Autodesk Inventor part; units mm, degrees
(part 4 of 4)
sketch "Двотавр 16" plane through (0, 0, 0) normal (0, 0, 1) x (1, 0, 0)
  arc A0 (264.3183, 276.423) -> (256.8007, 284.866) centre (255.8183, 276.423) ccw
  arc A1 (276.8359, 284.866) -> (269.3183, 276.423) centre (277.8183, 276.423) ccw
  arc A2 (256.8007, 143.1381) -> (264.3183, 151.5811) centre (255.8183, 151.5811) ccw
  arc A3 (269.3183, 151.5811) -> (276.8359, 143.1381) centre (277.8183, 151.5811) ccw
  line L0 (226.3183, 134.002) -> (307.3183, 134.002)
  line L1 (269.3183, 151.5811) -> (269.3183, 276.423)
  line L2 (307.3183, 294.002) -> (226.3183, 294.002)
  line L3 (264.3183, 276.423) -> (264.3183, 151.5811)
  line L4 (276.8359, 284.866) -> (304.4882, 288.0835)
  arc A4 (304.4882, 288.0835) -> (307.3183, 291.262) centre (304.1183, 291.262) ccw
  line L5 (307.3183, 291.262) -> (307.3183, 294.002)
  line L6 (256.8007, 284.866) -> (229.1485, 288.0835)
  arc A5 (226.3183, 291.262) -> (229.1485, 288.0835) centre (229.5183, 291.262) ccw
  line L7 (226.3183, 291.262) -> (226.3183, 294.002)
  line L8 (256.8007, 143.1381) -> (229.1485, 139.9206)
  arc A6 (229.1485, 139.9206) -> (226.3183, 136.742) centre (229.5183, 136.742) ccw
  line L9 (226.3183, 136.742) -> (226.3183, 134.002)
  line L10 (307.3183, 134.002) -> (307.3183, 136.742)
  arc A7 (307.3183, 136.742) -> (304.4882, 139.9206) centre (304.1183, 136.742) ccw
  line L11 (304.4882, 139.9206) -> (276.8359, 143.1381)
  point P0 (262.5027, 203.4372)
  point P1 (266.8183, 294.002)
  point P2 (266.8183, 134.002)
  point P3 (288.3183, 141.802)
  dimension "d1065" = 160
  dimension "d1066" = 81
  dimension "d1067" = 5
  dimension "d1068" = 8.5
  dimension "d1069" = 3.2
  dimension "d1070" = 2.74
  dimension "d1071" = 19
  dimension "d1072" = 7.8
  measures "d1065" distance between parallel lines of L0 L2
  measures "d1066" distance of L0.start L0.end
  measures "d1067" distance between parallel lines of L3 L1
  measures "d1068" radius of A3
  measures "d1069" radius of A7
  measures "d1070" distance of L0.end L10.end
  measures "d1071" horizontal distance of L0.end point (288.318, 141.802)
  measures "d1072" distance from line of L0 point (288.318, 141.802)
sketch "Двотавр 18" plane through (0, 0, 0) normal (0, 0, 1) x (1, 0, 0)
  arc A0 (264.4171, 285.6439) -> (256.3127, 294.5993) centre (255.4171, 285.6439) ccw
  arc A1 (277.6216, 294.5993) -> (269.5171, 285.6439) centre (278.5171, 285.6439) ccw
  arc A2 (256.3127, 133.4234) -> (264.4171, 142.3788) centre (255.4171, 142.3788) ccw
  arc A3 (269.5171, 142.3788) -> (277.6216, 133.4234) centre (278.5171, 142.3788) ccw
  line L0 (221.9671, 124.0114) -> (311.9671, 124.0114)
  line L1 (269.5171, 142.3788) -> (269.5171, 285.6439)
  line L2 (311.9671, 304.0114) -> (221.9671, 304.0114)
  line L3 (264.4171, 285.6439) -> (264.4171, 142.3788)
  line L4 (277.6216, 294.5993) -> (308.8154, 297.7187)
  arc A4 (308.8154, 297.7187) -> (311.9671, 301.2014) centre (308.4671, 301.2014) ccw
  line L5 (311.9671, 301.2014) -> (311.9671, 304.0114)
  line L6 (256.3127, 294.5993) -> (225.1189, 297.7187)
  arc A5 (221.9671, 301.2014) -> (225.1189, 297.7187) centre (225.4671, 301.2014) ccw
  line L7 (221.9671, 301.2014) -> (221.9671, 304.0114)
  line L8 (256.3127, 133.4234) -> (225.1189, 130.304)
  arc A6 (225.1189, 130.304) -> (221.9671, 126.8214) centre (225.4671, 126.8214) ccw
  line L9 (221.9671, 126.8214) -> (221.9671, 124.0114)
  line L10 (311.9671, 124.0114) -> (311.9671, 126.8214)
  arc A7 (311.9671, 126.8214) -> (308.8154, 130.304) centre (308.4671, 126.8214) ccw
  line L11 (308.8154, 130.304) -> (277.6216, 133.4234)
  point P0 (262.5027, 203.4372)
  point P1 (266.9671, 304.0114)
  point P2 (266.9671, 124.0114)
  point P3 (290.7421, 132.1114)
  dimension "d1073" = 180
  dimension "d1074" = 90
  dimension "d1075" = 5.1
  dimension "d1076" = 9
  dimension "d1077" = 3.5
  dimension "d1078" = 2.81
  dimension "d1079" = 21.225
  dimension "d1080" = 8.1
  measures "d1073" distance between parallel lines of L0 L2
  measures "d1074" distance of L0.start L0.end
  measures "d1075" distance between parallel lines of L3 L1
  measures "d1076" radius of A3
  measures "d1077" radius of A7
  measures "d1078" distance of L0.end L10.end
  measures "d1079" horizontal distance of L0.end point (290.742, 132.111)
  measures "d1080" distance from line of L0 point (290.742, 132.111)
sketch "Двотавр 18а" plane through (0, 0, 0) normal (0, 0, 1) x (1, 0, 0)
  arc A0 (317.1236, 126.8284) -> (313.9635, 130.3118) centre (313.6236, 126.8284) ccw
  line L0 (313.9635, 130.3118) -> (277.7996, 133.8404)
  arc A1 (269.6736, 142.7979) -> (277.7996, 133.8404) centre (278.6736, 142.7979) ccw
  arc A2 (256.4476, 133.8404) -> (264.5736, 142.7979) centre (255.5736, 142.7979) ccw
  line L1 (217.1236, 124.0184) -> (317.1236, 124.0184)
  line L2 (256.4476, 133.8404) -> (220.2837, 130.3118)
  line L3 (217.1236, 126.8284) -> (217.1236, 124.0184)
  arc A3 (220.2837, 130.3118) -> (217.1236, 126.8284) centre (220.6236, 126.8284) ccw
  line L4 (269.6736, 142.7979) -> (269.6736, 285.2389)
  line L5 (264.5736, 285.2389) -> (264.5736, 142.7979)
  arc A4 (264.5736, 285.2389) -> (256.4476, 294.1964) centre (255.5736, 285.2389) ccw
  arc A5 (277.7996, 294.1964) -> (269.6736, 285.2389) centre (278.6736, 285.2389) ccw
  line L6 (256.4476, 294.1964) -> (220.2837, 297.7249)
  arc A6 (217.1236, 301.2084) -> (220.2837, 297.7249) centre (220.6236, 301.2084) ccw
  line L7 (317.1236, 304.0184) -> (217.1236, 304.0184)
  line L8 (217.1236, 301.2084) -> (217.1236, 304.0184)
  line L9 (277.7996, 294.1964) -> (313.9635, 297.7249)
  arc A7 (313.9635, 297.7249) -> (317.1236, 301.2084) centre (313.6236, 301.2084) ccw
  line L10 (317.1236, 301.2084) -> (317.1236, 304.0184)
  line L11 (317.1236, 124.0184) -> (317.1236, 126.8284)
  point P0 (262.5027, 203.4372)
  point P1 (293.3986, 132.3184)
  point P2 (267.1236, 124.0184)
  point P3 (267.1236, 304.0184)
  dimension "d1081" = 180
  dimension "d1082" = 100
  dimension "d1083" = 5.1
  dimension "d1084" = 9
  dimension "d1085" = 3.5
  dimension "d1086" = 2.81
  dimension "d1087" = 23.725
  dimension "d1088" = 8.3
  measures "d1081" distance between parallel lines of L1 L7
  measures "d1082" distance of L1.start L11.start
  measures "d1083" distance between parallel lines of L5 L4
  measures "d1084" radius of A1
  measures "d1085" radius of A0
  measures "d1086" distance of L11.start L11.end
  measures "d1087" horizontal distance of L11.start point (293.399, 132.318)
  measures "d1088" distance from line of L1 point (293.399, 132.318)
sketch "Двотавр 20" plane through (0, 0, 0) normal (0, 0, 1) x (1, 0, 0)
  arc A0 (317.1239, 116.4425) -> (313.522, 120.4227) centre (313.1239, 116.4425) ccw
  line L0 (313.522, 120.4227) -> (278.2786, 123.9471)
  arc A1 (269.7239, 133.4) -> (278.2786, 123.9471) centre (279.2239, 133.4) ccw
  arc A2 (255.9692, 123.9471) -> (264.5239, 133.4) centre (255.0239, 133.4) ccw
  line L1 (217.1239, 114.0325) -> (317.1239, 114.0325)
  line L2 (255.9692, 123.9471) -> (220.7259, 120.4227)
  line L3 (217.1239, 116.4425) -> (217.1239, 114.0325)
  arc A3 (220.7259, 120.4227) -> (217.1239, 116.4425) centre (221.1239, 116.4425) ccw
  line L4 (269.7239, 133.4) -> (269.7239, 294.6651)
  line L5 (264.5239, 294.6651) -> (264.5239, 133.4)
  arc A4 (264.5239, 294.6651) -> (255.9692, 304.118) centre (255.0239, 294.6651) ccw
  arc A5 (278.2786, 304.118) -> (269.7239, 294.6651) centre (279.2239, 294.6651) ccw
  line L6 (255.9692, 304.118) -> (220.7259, 307.6424)
  arc A6 (217.1239, 311.6225) -> (220.7259, 307.6424) centre (221.1239, 311.6225) ccw
  line L7 (317.1239, 314.0325) -> (217.1239, 314.0325)
  line L8 (217.1239, 311.6225) -> (217.1239, 314.0325)
  line L9 (278.2786, 304.118) -> (313.522, 307.6424)
  arc A7 (313.522, 307.6424) -> (317.1239, 311.6225) centre (313.1239, 311.6225) ccw
  line L10 (317.1239, 311.6225) -> (317.1239, 314.0325)
  line L11 (317.1239, 114.0325) -> (317.1239, 116.4425)
  point P0 (262.5027, 203.4372)
  point P1 (293.4239, 122.4325)
  point P2 (267.1239, 114.0325)
  point P3 (267.1239, 314.0325)
  dimension "d1089" = 200
  dimension "d1090" = 100
  dimension "d1091" = 5.2
  dimension "d1092" = 9.5
  dimension "d1093" = 4
  dimension "d1094" = 2.41
  dimension "d1095" = 23.7
  dimension "d1096" = 8.4
  measures "d1089" distance between parallel lines of L1 L7
  measures "d1090" distance of L1.start L11.start
  measures "d1091" distance between parallel lines of L5 L4
  measures "d1092" radius of A1
  measures "d1093" radius of A0
  measures "d1094" distance of L11.start L11.end
  measures "d1095" horizontal distance of L11.start point (293.424, 122.433)
  measures "d1096" distance from line of L1 point (293.424, 122.433)
sketch "Двотавр 20а" plane through (0, 0, 0) normal (0, 0, 1) x (1, 0, 0)
  line L0 (322.2804, 114.0395) -> (322.2804, 116.4495)
  arc A0 (322.2804, 116.4495) -> (318.6697, 120.4306) centre (318.2804, 116.4495) ccw
  line L1 (318.6697, 120.4306) -> (278.4558, 124.363)
  arc A1 (269.8804, 133.8179) -> (278.4558, 124.363) centre (279.3804, 133.8179) ccw
  arc A2 (256.1049, 124.363) -> (264.6804, 133.8179) centre (255.1804, 133.8179) ccw
  line L2 (212.2804, 114.0395) -> (322.2804, 114.0395)
  line L3 (256.1049, 124.363) -> (215.8911, 120.4306)
  line L4 (212.2804, 116.4495) -> (212.2804, 114.0395)
  arc A3 (215.8911, 120.4306) -> (212.2804, 116.4495) centre (216.2804, 116.4495) ccw
  line L5 (269.8804, 133.8179) -> (269.8804, 294.2612)
  line L6 (264.6804, 294.2612) -> (264.6804, 133.8179)
  line L7 (256.1049, 303.7161) -> (215.8911, 307.6485)
  arc A4 (212.2804, 311.6295) -> (215.8911, 307.6485) centre (216.2804, 311.6295) ccw
  line L8 (212.2804, 311.6295) -> (212.2804, 314.0395)
  line L9 (322.2804, 314.0395) -> (212.2804, 314.0395)
  arc A5 (264.6804, 294.2612) -> (256.1049, 303.7161) centre (255.1804, 294.2612) ccw
  arc A6 (278.4558, 303.7161) -> (269.8804, 294.2612) centre (279.3804, 294.2612) ccw
  line L10 (278.4558, 303.7161) -> (318.6697, 307.6485)
  line L11 (322.2804, 311.6295) -> (322.2804, 314.0395)
  arc A7 (318.6697, 307.6485) -> (322.2804, 311.6295) centre (318.2804, 311.6295) ccw
  point P0 (262.5027, 203.4372)
  point P1 (296.0804, 122.6395)
  point P2 (267.2804, 114.0395)
  point P3 (267.2804, 314.0395)
  dimension "d1097" = 200
  dimension "d1098" = 110
  dimension "d1099" = 5.2
  dimension "d1100" = 9.5
  dimension "d1101" = 4
  dimension "d1102" = 2.41
  dimension "d1103" = 26.2
  dimension "d1104" = 8.6
  measures "d1097" distance between parallel lines of L2 L9
  measures "d1098" distance of L2.start L0.start
  measures "d1099" distance between parallel lines of L6 L5
  measures "d1100" radius of A1
  measures "d1101" radius of A0
  measures "d1102" distance of L0.start L0.end
  measures "d1103" horizontal distance of L0.start point (296.08, 122.64)
  measures "d1104" distance from line of L2 point (296.08, 122.64)
sketch "Двотавр 22" plane through (0, 0, 0) normal (0, 0, 1) x (1, 0, 0)
  line L0 (322.294, 104.0391) -> (322.294, 106.5091)
  arc A0 (322.294, 106.5091) -> (318.6912, 110.4893) centre (318.294, 106.5091) ccw
  line L1 (318.6912, 110.4893) -> (279.0012, 114.4496)
  arc A1 (269.994, 124.4002) -> (279.0012, 114.4496) centre (279.994, 124.4002) ccw
  arc A2 (255.5869, 114.4496) -> (264.594, 124.4002) centre (254.594, 124.4002) ccw
  line L2 (212.294, 104.0391) -> (322.294, 104.0391)
  line L3 (255.5869, 114.4496) -> (215.8969, 110.4893)
  line L4 (212.294, 106.5091) -> (212.294, 104.0391)
  arc A3 (215.8969, 110.4893) -> (212.294, 106.5091) centre (216.294, 106.5091) ccw
  line L5 (269.994, 124.4002) -> (269.994, 303.678)
  line L6 (264.594, 303.678) -> (264.594, 124.4002)
  line L7 (255.5869, 313.6286) -> (215.8969, 317.5889)
  arc A4 (212.294, 321.5691) -> (215.8969, 317.5889) centre (216.294, 321.5691) ccw
  line L8 (212.294, 321.5691) -> (212.294, 324.0391)
  line L9 (322.294, 324.0391) -> (212.294, 324.0391)
  arc A5 (264.594, 303.678) -> (255.5869, 313.6286) centre (254.594, 303.678) ccw
  arc A6 (279.0012, 313.6286) -> (269.994, 303.678) centre (279.994, 303.678) ccw
  line L10 (279.0012, 313.6286) -> (318.6912, 317.5889)
  line L11 (322.294, 321.5691) -> (322.294, 324.0391)
  arc A7 (318.6912, 317.5889) -> (322.294, 321.5691) centre (318.294, 321.5691) ccw
  point P0 (262.5027, 203.4372)
  point P1 (296.144, 112.7391)
  point P2 (267.294, 104.0391)
  point P3 (267.294, 324.0391)
  dimension "d1105" = 220
  dimension "d1106" = 110
  dimension "d1107" = 5.4
  dimension "d1108" = 10
  dimension "d1109" = 4
  dimension "d1110" = 2.47
  dimension "d1111" = 26.15
  dimension "d1112" = 8.7
  measures "d1105" distance between parallel lines of L2 L9
  measures "d1106" distance of L2.start L0.start
  measures "d1107" distance between parallel lines of L6 L5
  measures "d1108" radius of A1
  measures "d1109" radius of A0
  measures "d1110" distance of L0.start L0.end
  measures "d1111" horizontal distance of L0.start point (296.144, 112.739)
  measures "d1112" distance from line of L2 point (296.144, 112.739)
sketch "Двотавр 22а" plane through (0, 0, 0) normal (0, 0, 1) x (1, 0, 0)
  line L0 (327.4505, 104.0461) -> (327.4505, 106.5161)
  arc A0 (327.4505, 106.5161) -> (323.8398, 110.4971) centre (323.4505, 106.5161) ccw
  line L1 (323.8398, 110.4971) -> (279.1771, 114.8654)
  arc A1 (270.1505, 124.8179) -> (279.1771, 114.8654) centre (280.1505, 124.8179) ccw
  arc A2 (255.7239, 114.8654) -> (264.7505, 124.8179) centre (254.7505, 124.8179) ccw
  line L2 (207.4505, 104.0461) -> (327.4505, 104.0461)
  line L3 (255.7239, 114.8654) -> (211.0611, 110.4971)
  line L4 (207.4505, 106.5161) -> (207.4505, 104.0461)
  arc A3 (211.0611, 110.4971) -> (207.4505, 106.5161) centre (211.4505, 106.5161) ccw
  line L5 (264.7505, 303.2743) -> (264.7505, 124.8179)
  line L6 (270.1505, 124.8179) -> (270.1505, 303.2743)
  line L7 (279.1771, 313.2268) -> (323.8398, 317.5951)
  arc A4 (323.8398, 317.5951) -> (327.4505, 321.5761) centre (323.4505, 321.5761) ccw
  line L8 (327.4505, 321.5761) -> (327.4505, 324.0461)
  line L9 (327.4505, 324.0461) -> (207.4505, 324.0461)
  arc A5 (279.1771, 313.2268) -> (270.1505, 303.2743) centre (280.1505, 303.2743) ccw
  arc A6 (264.7505, 303.2743) -> (255.7239, 313.2268) centre (254.7505, 303.2743) ccw
  line L10 (255.7239, 313.2268) -> (211.0611, 317.5951)
  arc A7 (207.4505, 321.5761) -> (211.0611, 317.5951) centre (211.4505, 321.5761) ccw
  line L11 (207.4505, 321.5761) -> (207.4505, 324.0461)
  point P0 (262.5027, 203.4372)
  point P1 (298.8005, 112.9461)
  point P2 (267.4505, 104.0461)
  point P3 (267.4505, 324.0461)
  dimension "d1113" = 220
  dimension "d1114" = 120
  dimension "d1115" = 5.4
  dimension "d1116" = 10
  dimension "d1117" = 4
  dimension "d1118" = 2.47
  dimension "d1119" = 28.65
  dimension "d1120" = 8.9
  measures "d1113" distance between parallel lines of L2 L9
  measures "d1114" distance of L2.start L0.start
  measures "d1115" distance between parallel lines of L5 L6
  measures "d1116" radius of A1
  measures "d1117" radius of A0
  measures "d1118" distance of L0.start L0.end
  measures "d1119" horizontal distance of L0.start point (298.8, 112.946)
  measures "d1120" distance from line of L2 point (298.8, 112.946)
sketch "Двотавр 24" plane through (0, 0, 0) normal (0, 0, 1) x (1, 0, 0)
  line L0 (264.5861, 312.3079) -> (264.5861, 115.7752)
  line L1 (270.1861, 115.7752) -> (270.1861, 312.3079)
  line L2 (279.6435, 322.7561) -> (321.2833, 326.9114)
  arc A0 (321.2833, 326.9114) -> (324.8861, 330.8916) centre (320.8861, 330.8916) ccw
  line L3 (324.8861, 330.8916) -> (324.8861, 334.0416)
  line L4 (324.8861, 334.0416) -> (209.8861, 334.0416)
  arc A1 (279.6435, 322.7561) -> (270.1861, 312.3079) centre (280.6861, 312.3079) ccw
  arc A2 (264.5861, 312.3079) -> (255.1288, 322.7561) centre (254.0861, 312.3079) ccw
  line L5 (255.1288, 322.7561) -> (213.4889, 326.9114)
  arc A3 (209.8861, 330.8916) -> (213.4889, 326.9114) centre (213.8861, 330.8916) ccw
  line L6 (209.8861, 330.8916) -> (209.8861, 334.0416)
  line L7 (324.8861, 94.0416) -> (324.8861, 97.1916)
  arc A4 (324.8861, 97.1916) -> (321.2833, 101.1718) centre (320.8861, 97.1916) ccw
  line L8 (321.2833, 101.1718) -> (279.6435, 105.3271)
  arc A5 (255.1288, 105.3271) -> (264.5861, 115.7752) centre (254.0861, 115.7752) ccw
  line L9 (209.8861, 94.0416) -> (324.8861, 94.0416)
  arc A6 (270.1861, 115.7752) -> (279.6435, 105.3271) centre (280.6861, 115.7752) ccw
  line L10 (255.1288, 105.3271) -> (213.4889, 101.1718)
  arc A7 (213.4889, 101.1718) -> (209.8861, 97.1916) centre (213.8861, 97.1916) ccw
  line L11 (209.8861, 97.1916) -> (209.8861, 94.0416)
  point P0 (262.5027, 203.4372)
  point P1 (267.3861, 334.0416)
  point P2 (297.5361, 103.5416)
  point P3 (267.3861, 94.0416)
  dimension "d1121" = 240
  dimension "d1122" = 115
  dimension "d1123" = 5.6
  dimension "d1124" = 10.5
  dimension "d1125" = 4
  dimension "d1126" = 3.15
  dimension "d1127" = 27.35
  dimension "d1128" = 9.5
  measures "d1121" distance between parallel lines of L9 L4
  measures "d1122" distance of L9.start L9.end
  measures "d1123" distance between parallel lines of L0 L1
  measures "d1124" radius of A6
  measures "d1125" radius of A4
  measures "d1126" distance of L9.end L7.end
  measures "d1127" horizontal distance of L9.end point (297.536, 103.542)
  measures "d1128" distance from line of L9 point (297.536, 103.542)
sketch "Двотавр 24а" plane through (0, 0, 0) normal (0, 0, 1) x (1, 0, 0)
  line L0 (255.3043, 105.9275) -> (208.637, 101.1807)
  arc A0 (208.637, 101.1807) -> (205.0418, 97.2013) centre (209.0418, 97.2013) ccw
  line L1 (205.0418, 94.0513) -> (330.0418, 94.0513)
  line L2 (205.0418, 97.2013) -> (205.0418, 94.0513)
  arc A1 (255.3043, 105.9275) -> (264.7418, 116.3736) centre (254.2418, 116.3736) ccw
  arc A2 (270.3418, 116.3736) -> (279.7793, 105.9275) centre (280.8418, 116.3736) ccw
  line L3 (326.4466, 101.1807) -> (279.7793, 105.9275)
  line L4 (330.0418, 94.0513) -> (330.0418, 97.2013)
  arc A3 (330.0418, 97.2013) -> (326.4466, 101.1807) centre (326.0418, 97.2013) ccw
  line L5 (264.7418, 311.7289) -> (264.7418, 116.3736)
  line L6 (270.3418, 116.3736) -> (270.3418, 311.7289)
  line L7 (279.7793, 322.175) -> (326.4466, 326.9218)
  arc A4 (326.4466, 326.9218) -> (330.0418, 330.9013) centre (326.0418, 330.9013) ccw
  line L8 (330.0418, 330.9013) -> (330.0418, 334.0513)
  arc A5 (279.7793, 322.175) -> (270.3418, 311.7289) centre (280.8418, 311.7289) ccw
  arc A6 (264.7418, 311.7289) -> (255.3043, 322.175) centre (254.2418, 311.7289) ccw
  line L9 (330.0418, 334.0513) -> (205.0418, 334.0513)
  line L10 (255.3043, 322.175) -> (208.637, 326.9218)
  arc A7 (205.0418, 330.9013) -> (208.637, 326.9218) centre (209.0418, 330.9013) ccw
  line L11 (205.0418, 330.9013) -> (205.0418, 334.0513)
  point P0 (262.5027, 203.4372)
  point P1 (267.5418, 94.0513)
  point P2 (300.1918, 103.8513)
  point P3 (267.5418, 334.0513)
  dimension "d1129" = 240
  dimension "d1130" = 125
  dimension "d1131" = 5.6
  dimension "d1132" = 10.5
  dimension "d1133" = 4
  dimension "d1134" = 3.15
  dimension "d1135" = 29.85
  dimension "d1136" = 9.8
  measures "d1129" distance between parallel lines of L1 L9
  measures "d1130" distance of L1.start L1.end
  measures "d1131" distance between parallel lines of L5 L6
  measures "d1132" radius of A2
  measures "d1133" radius of A3
  measures "d1134" distance of L1.end L4.end
  measures "d1135" horizontal distance of L1.end point (300.192, 103.851)
  measures "d1136" distance from line of L1 point (300.192, 103.851)
sketch "Двотавр 27" plane through (0, 0, 0) normal (0, 0, 1) x (1, 0, 0)
  line L0 (254.6336, 90.843) -> (209.0957, 86.3024)
  arc A0 (209.0957, 86.3024) -> (205.0422, 81.8246) centre (209.5422, 81.8246) ccw
  line L1 (205.0422, 79.0646) -> (330.0422, 79.0646)
  line L2 (205.0422, 81.8246) -> (205.0422, 79.0646)
  arc A1 (254.6336, 90.843) -> (264.5422, 101.7887) centre (253.5422, 101.7887) ccw
  arc A2 (270.5422, 101.7887) -> (280.4508, 90.843) centre (281.5422, 101.7887) ccw
  line L3 (325.9887, 86.3024) -> (280.4508, 90.843)
  line L4 (330.0422, 79.0646) -> (330.0422, 81.8246)
  arc A3 (330.0422, 81.8246) -> (325.9887, 86.3024) centre (325.5422, 81.8246) ccw
  line L5 (264.5422, 326.3405) -> (264.5422, 101.7887)
  line L6 (270.5422, 101.7887) -> (270.5422, 326.3405)
  line L7 (280.4508, 337.2862) -> (325.9887, 341.8268)
  arc A4 (325.9887, 341.8268) -> (330.0422, 346.3046) centre (325.5422, 346.3046) ccw
  line L8 (330.0422, 346.3046) -> (330.0422, 349.0646)
  arc A5 (280.4508, 337.2862) -> (270.5422, 326.3405) centre (281.5422, 326.3405) ccw
  arc A6 (264.5422, 326.3405) -> (254.6336, 337.2862) centre (253.5422, 326.3405) ccw
  line L9 (330.0422, 349.0646) -> (205.0422, 349.0646)
  line L10 (254.6336, 337.2862) -> (209.0957, 341.8268)
  arc A7 (205.0422, 346.3046) -> (209.0957, 341.8268) centre (209.5422, 346.3046) ccw
  line L11 (205.0422, 346.3046) -> (205.0422, 349.0646)
  point P0 (262.5027, 203.4372)
  point P1 (267.5422, 79.0646)
  point P2 (300.2922, 88.8646)
  point P3 (267.5422, 349.0646)
  dimension "d1137" = 270
  dimension "d1138" = 125
  dimension "d1139" = 6
  dimension "d1140" = 11
  dimension "d1141" = 4.5
  dimension "d1142" = 2.76
  dimension "d1143" = 29.75
  dimension "d1144" = 9.8
  measures "d1137" distance between parallel lines of L1 L9
  measures "d1138" distance of L1.start L1.end
  measures "d1139" distance between parallel lines of L5 L6
  measures "d1140" radius of A2
  measures "d1141" radius of A3
  measures "d1142" distance of L1.end L4.end
  measures "d1143" horizontal distance of L1.end point (300.292, 88.865)
  measures "d1144" distance from line of L1 point (300.292, 88.865)
sketch "Двотавр 27а" plane through (0, 0, 0) normal (0, 0, 1) x (1, 0, 0)
  line L0 (254.8464, 91.6302) -> (204.227, 86.3124)
  arc A0 (204.227, 86.3124) -> (200.1971, 81.8371) centre (204.6971, 81.8371) ccw
  line L1 (200.1971, 79.0771) -> (335.1971, 79.0771)
  line L2 (200.1971, 81.8371) -> (200.1971, 79.0771)
  arc A1 (254.8464, 91.6302) -> (264.6971, 102.57) centre (253.6971, 102.57) ccw
  arc A2 (270.6971, 102.57) -> (280.5479, 91.6302) centre (281.6971, 102.57) ccw
  line L3 (331.1673, 86.3124) -> (280.5479, 91.6302)
  arc A3 (335.1971, 81.8371) -> (331.1673, 86.3124) centre (330.6971, 81.8371) ccw
  line L4 (335.1971, 79.0771) -> (335.1971, 81.8371)
  line L5 (270.6971, 102.57) -> (270.6971, 325.5841)
  line L6 (264.6971, 325.5841) -> (264.6971, 102.57)
  arc A4 (280.5479, 336.5239) -> (270.6971, 325.5841) centre (281.6971, 325.5841) ccw
  line L7 (280.5479, 336.5239) -> (331.1673, 341.8417)
  arc A5 (331.1673, 341.8417) -> (335.1971, 346.3171) centre (330.6971, 346.3171) ccw
  line L8 (335.1971, 346.3171) -> (335.1971, 349.0771)
  line L9 (335.1971, 349.0771) -> (200.1971, 349.0771)
  line L10 (254.8464, 336.5239) -> (204.227, 341.8417)
  arc A6 (200.1971, 346.3171) -> (204.227, 341.8417) centre (204.6971, 346.3171) ccw
  line L11 (200.1971, 346.3171) -> (200.1971, 349.0771)
  arc A7 (264.6971, 325.5841) -> (254.8464, 336.5239) centre (253.6971, 325.5841) ccw
  point P0 (262.5027, 203.4372)
  point P1 (267.6971, 79.0771)
  point P2 (302.9471, 89.2771)
  point P3 (267.6971, 349.0771)
  dimension "d1153" = 270
  dimension "d1154" = 135
  dimension "d1155" = 6
  dimension "d1156" = 11
  dimension "d1157" = 4.5
  dimension "d1158" = 2.76
  dimension "d1159" = 32.25
  dimension "d1160" = 10.2
  measures "d1153" distance between parallel lines of L1 L9
  measures "d1154" distance of L1.start L4.start
  measures "d1155" distance between parallel lines of L6 L5
  measures "d1156" radius of A2
  measures "d1157" radius of A3
  measures "d1158" distance of L4.start L4.end
  measures "d1159" horizontal distance of L4.start point (302.947, 89.277)
  measures "d1160" distance from line of L1 point (302.947, 89.277)
sketch "Двотавр 30" plane through (0, 0, 0) normal (0, 0, 1) x (1, 0, 0)
  line L0 (253.6531, 76.412) -> (204.7161, 71.5315)
  arc A0 (204.7161, 71.5315) -> (200.2123, 66.5562) centre (205.2123, 66.5562) ccw
  line L1 (200.2123, 64.0862) -> (335.2123, 64.0862)
  line L2 (200.2123, 66.5562) -> (200.2123, 64.0862)
  arc A1 (253.6531, 76.412) -> (264.4623, 88.3528) centre (252.4623, 88.3528) ccw
  arc A2 (270.9623, 88.3528) -> (281.7714, 76.412) centre (282.9623, 88.3528) ccw
  line L3 (330.7085, 71.5315) -> (281.7714, 76.412)
  arc A3 (335.2123, 66.5562) -> (330.7085, 71.5315) centre (330.2123, 66.5562) ccw
  line L4 (335.2123, 64.0862) -> (335.2123, 66.5562)
  line L5 (270.9623, 88.3528) -> (270.9623, 339.8196)
  line L6 (264.4623, 339.8196) -> (264.4623, 88.3528)
  arc A4 (281.7714, 351.7603) -> (270.9623, 339.8196) centre (282.9623, 339.8196) ccw
  line L7 (281.7714, 351.7603) -> (330.7085, 356.6408)
  arc A5 (330.7085, 356.6408) -> (335.2123, 361.6162) centre (330.2123, 361.6162) ccw
  line L8 (335.2123, 361.6162) -> (335.2123, 364.0862)
  line L9 (335.2123, 364.0862) -> (200.2123, 364.0862)
  line L10 (253.6531, 351.7603) -> (204.7161, 356.6408)
  arc A6 (200.2123, 361.6162) -> (204.7161, 356.6408) centre (205.2123, 361.6162) ccw
  line L11 (200.2123, 361.6162) -> (200.2123, 364.0862)
  arc A7 (264.4623, 339.8196) -> (253.6531, 351.7603) centre (252.4623, 339.8196) ccw
  point P0 (262.5027, 203.4372)
  point P1 (267.7123, 64.0862)
  point P2 (303.0873, 74.2862)
  point P3 (267.7123, 364.0862)
  dimension "d1161" = 300
  dimension "d1162" = 135
  dimension "d1163" = 6.5
  dimension "d1164" = 12
  dimension "d1165" = 5
  dimension "d1166" = 2.47
  dimension "d1167" = 32.125
  dimension "d1168" = 10.2
  measures "d1161" distance between parallel lines of L1 L9
  measures "d1162" distance of L1.start L4.start
  measures "d1163" distance between parallel lines of L6 L5
  measures "d1164" radius of A2
  measures "d1165" radius of A3
  measures "d1166" distance of L4.start L4.end
  measures "d1167" horizontal distance of L4.start point (303.087, 74.286)
  measures "d1168" distance from line of L1 point (303.087, 74.286)
sketch "Двотавр 30а" plane through (0, 0, 0) normal (0, 0, 1) x (1, 0, 0)
  line L0 (340.3665, 64.1013) -> (340.3665, 66.5713)
  arc A0 (340.3665, 66.5713) -> (335.9036, 71.5424) centre (335.3665, 66.5713) ccw
  arc A1 (281.8275, 350.8175) -> (271.1165, 338.8869) centre (283.1165, 338.8869) ccw
  arc A2 (264.6165, 338.8869) -> (253.9056, 350.8175) centre (252.6165, 338.8869) ccw
  line L1 (281.8275, 350.8175) -> (335.9036, 356.6602)
  arc A3 (335.9036, 356.6602) -> (340.3665, 361.6313) centre (335.3665, 361.6313) ccw
  line L2 (340.3665, 361.6313) -> (340.3665, 364.1013)
  line L3 (340.3665, 364.1013) -> (195.3665, 364.1013)
  line L4 (253.9056, 350.8175) -> (199.8294, 356.6602)
  arc A4 (195.3665, 361.6313) -> (199.8294, 356.6602) centre (200.3665, 361.6313) ccw
  line L5 (195.3665, 361.6313) -> (195.3665, 364.1013)
  line L6 (335.9036, 71.5424) -> (281.8275, 77.3852)
  arc A5 (271.1165, 89.3157) -> (281.8275, 77.3852) centre (283.1165, 89.3157) ccw
  arc A6 (253.9056, 77.3852) -> (264.6165, 89.3157) centre (252.6165, 89.3157) ccw
  line L7 (195.3665, 64.1013) -> (340.3665, 64.1013)
  line L8 (253.9056, 77.3852) -> (199.8294, 71.5424)
  line L9 (195.3665, 66.5713) -> (195.3665, 64.1013)
  arc A7 (199.8294, 71.5424) -> (195.3665, 66.5713) centre (200.3665, 66.5713) ccw
  line L10 (271.1165, 89.3157) -> (271.1165, 338.8869)
  line L11 (264.6165, 338.8869) -> (264.6165, 89.3157)
  point P0 (262.5027, 203.4372)
  point P1 (267.8665, 364.1013)
  point P2 (305.7415, 74.8013)
  point P3 (267.8665, 64.1013)
  dimension "d1169" = 300
  dimension "d1170" = 145
  dimension "d1171" = 6.5
  dimension "d1172" = 12
  dimension "d1173" = 5
  dimension "d1174" = 2.47
  dimension "d1175" = 34.625
  dimension "d1176" = 10.7
  measures "d1169" distance between parallel lines of L7 L3
  measures "d1170" distance of L7.start L0.start
  measures "d1171" distance between parallel lines of L11 L10
  measures "d1172" radius of A5
  measures "d1173" radius of A0
  measures "d1174" distance of L0.start L0.end
  measures "d1175" horizontal distance of L0.start point (305.742, 74.801)
  measures "d1176" distance from line of L7 point (305.742, 74.801)
sketch "Двотавр 33" plane through (0, 0, 0) normal (0, 0, 1) x (1, 0, 0)
  line L0 (337.8184, 49.0868) -> (337.8184, 52.4468)
  arc A0 (337.8184, 52.4468) -> (333.3142, 57.4222) centre (332.8184, 52.4468) ccw
  arc A1 (283.0293, 365.7404) -> (271.3184, 352.8045) centre (284.3184, 352.8045) ccw
  arc A2 (264.3184, 352.8045) -> (252.6075, 365.7404) centre (251.3184, 352.8045) ccw
  line L1 (283.0293, 365.7404) -> (333.3142, 370.7515)
  arc A3 (333.3142, 370.7515) -> (337.8184, 375.7268) centre (332.8184, 375.7268) ccw
  line L2 (337.8184, 375.7268) -> (337.8184, 379.0868)
  line L3 (337.8184, 379.0868) -> (197.8184, 379.0868)
  line L4 (252.6075, 365.7404) -> (202.3226, 370.7515)
  arc A4 (197.8184, 375.7268) -> (202.3226, 370.7515) centre (202.8184, 375.7268) ccw
  line L5 (197.8184, 375.7268) -> (197.8184, 379.0868)
  line L6 (333.3142, 57.4222) -> (283.0293, 62.4333)
  arc A5 (271.3184, 75.3692) -> (283.0293, 62.4333) centre (284.3184, 75.3692) ccw
  arc A6 (252.6075, 62.4333) -> (264.3184, 75.3692) centre (251.3184, 75.3692) ccw
  line L7 (197.8184, 49.0868) -> (337.8184, 49.0868)
  line L8 (252.6075, 62.4333) -> (202.3226, 57.4222)
  line L9 (197.8184, 52.4468) -> (197.8184, 49.0868)
  arc A7 (202.3226, 57.4222) -> (197.8184, 52.4468) centre (202.8184, 52.4468) ccw
  line L10 (271.3184, 75.3692) -> (271.3184, 352.8045)
  line L11 (264.3184, 352.8045) -> (264.3184, 75.3692)
  point P0 (262.5027, 203.4372)
  point P1 (267.8184, 379.0868)
  point P2 (304.5684, 60.2868)
  point P3 (267.8184, 49.0868)
  dimension "d1177" = 330
  dimension "d1178" = 140
  dimension "d1179" = 7
  dimension "d1180" = 13
  dimension "d1181" = 5
  dimension "d1182" = 3.36
  dimension "d1183" = 33.25
  dimension "d1184" = 11.2
  measures "d1177" distance between parallel lines of L7 L3
  measures "d1178" distance of L7.start L0.start
  measures "d1179" distance between parallel lines of L11 L10
  measures "d1180" radius of A5
  measures "d1181" radius of A0
  measures "d1182" distance of L0.start L0.end
  measures "d1183" horizontal distance of L0.start point (304.568, 60.287)
  measures "d1184" distance from line of L7 point (304.568, 60.287)
sketch "Двотавр 36" plane through (0, 0, 0) normal (0, 0, 1) x (1, 0, 0)
  line L0 (340.3964, 34.1209) -> (340.3964, 37.5609)
  arc A0 (340.3964, 37.5609) -> (334.9919, 43.5312) centre (334.3964, 37.5609) ccw
  arc A1 (284.2568, 379.65) -> (271.6464, 365.7191) centre (285.6464, 365.7191) ccw
  arc A2 (264.1464, 365.7191) -> (251.5359, 379.65) centre (250.1464, 365.7191) ccw
  line L1 (284.2568, 379.65) -> (334.9919, 384.7105)
  arc A3 (334.9919, 384.7105) -> (340.3964, 390.6809) centre (334.3964, 390.6809) ccw
  line L2 (340.3964, 390.6809) -> (340.3964, 394.1209)
  line L3 (340.3964, 394.1209) -> (195.3964, 394.1209)
  line L4 (251.5359, 379.65) -> (200.8009, 384.7105)
  arc A4 (195.3964, 390.6809) -> (200.8009, 384.7105) centre (201.3964, 390.6809) ccw
  line L5 (195.3964, 390.6809) -> (195.3964, 394.1209)
  line L6 (334.9919, 43.5312) -> (284.2568, 48.5917)
  arc A5 (271.6464, 62.5226) -> (284.2568, 48.5917) centre (285.6464, 62.5226) ccw
  arc A6 (251.5359, 48.5917) -> (264.1464, 62.5226) centre (250.1464, 62.5226) ccw
  line L7 (195.3964, 34.1209) -> (340.3964, 34.1209)
  line L8 (251.5359, 48.5917) -> (200.8009, 43.5312)
  line L9 (195.3964, 37.5609) -> (195.3964, 34.1209)
  arc A7 (200.8009, 43.5312) -> (195.3964, 37.5609) centre (201.3964, 37.5609) ccw
  line L10 (271.6464, 62.5226) -> (271.6464, 365.7191)
  line L11 (264.1464, 365.7191) -> (264.1464, 62.5226)
  point P0 (262.5027, 203.4372)
  point P1 (267.8964, 394.1209)
  point P2 (306.0214, 46.4209)
  point P3 (267.8964, 34.1209)
  dimension "d1185" = 360
  dimension "d1186" = 145
  dimension "d1187" = 7.5
  dimension "d1188" = 14
  dimension "d1189" = 6
  dimension "d1190" = 3.44
  dimension "d1191" = 34.375
  dimension "d1192" = 12.3
  measures "d1185" distance between parallel lines of L7 L3
  measures "d1186" distance of L7.start L0.start
  measures "d1187" distance between parallel lines of L11 L10
  measures "d1188" radius of A5
  measures "d1189" radius of A0
  measures "d1190" distance of L0.start L0.end
  measures "d1191" horizontal distance of L0.start point (306.021, 46.421)
  measures "d1192" distance from line of L7 point (306.021, 46.421)
sketch "Двотавр 40" plane through (0, 0, 0) normal (0, 0, 1) x (1, 0, 0)
  line L0 (345.5809, 14.1255) -> (345.5809, 18.0355)
  arc A0 (345.5809, 18.0355) -> (340.1765, 24.0059) centre (339.5809, 18.0355) ccw
  arc A1 (285.7418, 398.8146) -> (272.2309, 383.8887) centre (287.2309, 383.8887) ccw
  arc A2 (263.9309, 383.8887) -> (250.4199, 398.8146) centre (248.9309, 383.8887) ccw
  line L1 (285.7418, 398.8146) -> (340.1765, 404.2451)
  arc A3 (340.1765, 404.2451) -> (345.5809, 410.2155) centre (339.5809, 410.2155) ccw
  line L2 (345.5809, 410.2155) -> (345.5809, 414.1255)
  line L3 (345.5809, 414.1255) -> (190.5809, 414.1255)
  line L4 (250.4199, 398.8146) -> (195.9852, 404.2451)
  arc A4 (190.5809, 410.2155) -> (195.9852, 404.2451) centre (196.5809, 410.2155) ccw
  line L5 (190.5809, 410.2155) -> (190.5809, 414.1255)
  line L6 (340.1765, 24.0059) -> (285.7418, 29.4364)
  arc A5 (272.2309, 44.3623) -> (285.7418, 29.4364) centre (287.2309, 44.3623) ccw
  arc A6 (250.4199, 29.4364) -> (263.9309, 44.3623) centre (248.9309, 44.3623) ccw
  line L7 (190.5809, 14.1255) -> (345.5809, 14.1255)
  line L8 (250.4199, 29.4364) -> (195.9852, 24.0059)
  line L9 (190.5809, 18.0355) -> (190.5809, 14.1255)
  arc A7 (195.9852, 24.0059) -> (190.5809, 18.0355) centre (196.5809, 18.0355) ccw
  line L10 (272.2309, 44.3623) -> (272.2309, 383.8887)
  line L11 (263.9309, 383.8887) -> (263.9309, 44.3623)
  point P0 (262.5027, 203.4372)
  point P1 (268.0809, 414.1255)
  point P2 (308.9059, 27.1255)
  point P3 (268.0809, 14.1255)
  dimension "d1193" = 400
  dimension "d1194" = 155
  dimension "d1195" = 8.3
  dimension "d1196" = 15
  dimension "d1197" = 6
  dimension "d1198" = 3.91
  dimension "d1199" = 36.675
  dimension "d1200" = 13
  measures "d1193" distance between parallel lines of L7 L3
  measures "d1194" distance of L7.start L0.start
  measures "d1195" distance between parallel lines of L11 L10
  measures "d1196" radius of A5
  measures "d1197" radius of A0
  measures "d1198" distance of L0.start L0.end
  measures "d1199" horizontal distance of L0.start point (308.906, 27.125)
  measures "d1200" distance from line of L7 point (308.906, 27.125)
sketch "Двотавр 45" plane through (0, 0, 0) normal (0, 0, 1) x (1, 0, 0)
  line L0 (348.1589, -10.8408) -> (348.1589, -6.7408)
  arc A0 (287.0718, 422.6329) -> (272.6589, 406.7118) centre (288.6589, 406.7118) ccw
  arc A1 (263.6589, 406.7118) -> (249.246, 422.6329) centre (247.6589, 406.7118) ccw
  line L1 (287.0718, 422.6329) -> (341.8533, 428.0937)
  arc A2 (341.8533, 428.0937) -> (348.1589, 435.0592) centre (341.1589, 435.0592) ccw
  line L2 (348.1589, 435.0592) -> (348.1589, 439.1592)
  line L3 (348.1589, 439.1592) -> (188.1589, 439.1592)
  line L4 (249.246, 422.6329) -> (194.4645, 428.0937)
  arc A3 (188.1589, 435.0592) -> (194.4645, 428.0937) centre (195.1589, 435.0592) ccw
  line L5 (188.1589, 435.0592) -> (188.1589, 439.1592)
  arc A4 (348.1589, -6.7408) -> (341.8533, 0.2247) centre (341.1589, -6.7408) ccw
  line L6 (341.8533, 0.2247) -> (287.0718, 5.6856)
  arc A5 (272.6589, 21.6067) -> (287.0718, 5.6856) centre (288.6589, 21.6067) ccw
  arc A6 (249.246, 5.6856) -> (263.6589, 21.6067) centre (247.6589, 21.6067) ccw
  line L7 (188.1589, -10.8408) -> (348.1589, -10.8408)
  line L8 (188.1589, -6.7408) -> (188.1589, -10.8408)
  arc A7 (194.4645, 0.2247) -> (188.1589, -6.7408) centre (195.1589, -6.7408) ccw
  line L9 (272.6589, 21.6067) -> (272.6589, 406.7118)
  line L10 (263.6589, 406.7118) -> (263.6589, 21.6067)
  line L11 (249.246, 5.6856) -> (194.4645, 0.2247)
  point P0 (262.5027, 203.4372)
  point P1 (268.1589, 439.1592)
  point P2 (310.4089, 3.3592)
  point P3 (268.1589, -10.8408)
  dimension "d1201" = 450
  dimension "d1202" = 160
  dimension "d1203" = 9
  dimension "d1204" = 16
  dimension "d1205" = 7
  dimension "d1206" = 4.1
  dimension "d1207" = 37.75
  dimension "d1208" = 14.2
  measures "d1201" distance between parallel lines of L7 L3
  measures "d1202" distance of L8.end L0.start
  measures "d1203" distance between parallel lines of L10 L9
  measures "d1204" radius of A5
  measures "d1205" radius of A4
  measures "d1206" distance of L0.start L0.end
  measures "d1207" horizontal distance of L0.start point (310.409, 3.359)
  measures "d1208" distance from line of L7 point (310.409, 3.359)
sketch "Двотавр 50" plane through (0, 0, 0) normal (0, 0, 1) x (1, 0, 0)
  line L0 (353.3429, -35.8362) -> (353.3429, -30.9662)
  arc A0 (288.6538, 446.4985) -> (273.3429, 429.5827) centre (290.3429, 429.5827) ccw
  arc A1 (263.3429, 429.5827) -> (248.032, 446.4985) centre (246.3429, 429.5827) ccw
  line L1 (288.6538, 446.4985) -> (347.0384, 452.3285)
  arc A2 (347.0384, 452.3285) -> (353.3429, 459.2938) centre (346.3429, 459.2938) ccw
  line L2 (353.3429, 459.2938) -> (353.3429, 464.1638)
  line L3 (353.3429, 464.1638) -> (183.3429, 464.1638)
  line L4 (248.032, 446.4985) -> (189.6474, 452.3285)
  arc A3 (183.3429, 459.2938) -> (189.6474, 452.3285) centre (190.3429, 459.2938) ccw
  line L5 (183.3429, 459.2938) -> (183.3429, 464.1638)
  arc A4 (353.3429, -30.9662) -> (347.0384, -24.0008) centre (346.3429, -30.9662) ccw
  line L6 (347.0384, -24.0008) -> (288.6538, -18.1708)
  arc A5 (273.3429, -1.255) -> (288.6538, -18.1708) centre (290.3429, -1.255) ccw
  arc A6 (248.032, -18.1708) -> (263.3429, -1.255) centre (246.3429, -1.255) ccw
  line L7 (183.3429, -35.8362) -> (353.3429, -35.8362)
  line L8 (183.3429, -30.9662) -> (183.3429, -35.8362)
  arc A7 (189.6474, -24.0008) -> (183.3429, -30.9662) centre (190.3429, -30.9662) ccw
  line L9 (273.3429, -1.255) -> (273.3429, 429.5827)
  line L10 (263.3429, 429.5827) -> (263.3429, -1.255)
  line L11 (248.032, -18.1708) -> (189.6474, -24.0008)
  point P0 (262.5027, 203.4372)
  point P1 (268.3429, 464.1638)
  point P2 (313.3429, -20.6362)
  point P3 (268.3429, -35.8362)
  dimension "d1209" = 500
  dimension "d1210" = 170
  dimension "d1211" = 10
  dimension "d1212" = 17
  dimension "d1213" = 7
  dimension "d1214" = 4.87
  dimension "d1215" = 40
  dimension "d1216" = 15.2
  measures "d1209" distance between parallel lines of L7 L3
  measures "d1210" distance of L8.end L0.start
  measures "d1211" distance between parallel lines of L10 L9
  measures "d1212" radius of A5
  measures "d1213" radius of A4
  measures "d1214" distance of L0.start L0.end
  measures "d1215" horizontal distance of L0.start point (313.343, -20.636)
  measures "d1216" distance from line of L7 point (313.343, -20.636)
sketch "Двотавр 55" plane through (0, 0, 0) normal (0, 0, 1) x (1, 0, 0)
  line L0 (358.5274, -60.8318) -> (358.5274, -54.8818)
  arc A0 (290.2413, 470.0717) -> (274.0274, 452.1606) centre (292.0274, 452.1606) ccw
  arc A1 (263.0274, 452.1606) -> (246.8136, 470.0717) centre (245.0274, 452.1606) ccw
  line L1 (290.2413, 470.0717) -> (352.2221, 476.2527)
  arc A2 (352.2221, 476.2527) -> (358.5274, 483.2182) centre (351.5274, 483.2182) ccw
  line L2 (358.5274, 483.2182) -> (358.5274, 489.1682)
  line L3 (358.5274, 489.1682) -> (178.5274, 489.1682)
  line L4 (246.8136, 470.0717) -> (184.8328, 476.2527)
  arc A3 (178.5274, 483.2182) -> (184.8328, 476.2527) centre (185.5274, 483.2182) ccw
  line L5 (178.5274, 483.2182) -> (178.5274, 489.1682)
  arc A4 (358.5274, -54.8818) -> (352.2221, -47.9164) centre (351.5274, -54.8818) ccw
  line L6 (352.2221, -47.9164) -> (290.2413, -41.7354)
  arc A5 (274.0274, -23.8242) -> (290.2413, -41.7354) centre (292.0274, -23.8242) ccw
  arc A6 (246.8136, -41.7354) -> (263.0274, -23.8242) centre (245.0274, -23.8242) ccw
  line L7 (178.5274, -60.8318) -> (358.5274, -60.8318)
  line L8 (178.5274, -54.8818) -> (178.5274, -60.8318)
  arc A7 (184.8328, -47.9164) -> (178.5274, -54.8818) centre (185.5274, -54.8818) ccw
  line L9 (274.0274, -23.8242) -> (274.0274, 452.1606)
  line L10 (263.0274, 452.1606) -> (263.0274, -23.8242)
  line L11 (246.8136, -41.7354) -> (184.8328, -47.9164)
  point P0 (262.5027, 203.4372)
  point P1 (268.5274, 489.1682)
  point P2 (316.2774, -44.3318)
  point P3 (268.5274, -60.8318)
  dimension "d1217" = 550
  dimension "d1218" = 180
  dimension "d1219" = 11
  dimension "d1220" = 18
  dimension "d1221" = 7
  dimension "d1222" = 5.95
  dimension "d1223" = 42.25
  dimension "d1224" = 16.5
  measures "d1217" distance between parallel lines of L7 L3
  measures "d1218" distance of L8.end L0.start
  measures "d1219" distance between parallel lines of L10 L9
  measures "d1220" radius of A5
  measures "d1221" radius of A4
  measures "d1222" distance of L0.start L0.end
  measures "d1223" horizontal distance of L0.start point (316.277, -44.332)
  measures "d1224" distance from line of L7 point (316.277, -44.332)
sketch "Двотавр 60" plane through (0, 0, 0) normal (0, 0, 1) x (1, 0, 0)
  line L0 (363.7104, -85.7971) -> (363.7104, -79.6771)
  arc A0 (292.7256, 493.7615) -> (274.7104, 473.8602) centre (294.7104, 473.8602) ccw
  arc A1 (262.7104, 473.8602) -> (244.6953, 493.7615) centre (242.7104, 473.8602) ccw
  line L1 (292.7256, 493.7615) -> (356.5044, 500.1224)
  arc A2 (356.5044, 500.1224) -> (363.7104, 508.0829) centre (355.7104, 508.0829) ccw
  line L2 (363.7104, 508.0829) -> (363.7104, 514.2029)
  line L3 (363.7104, 514.2029) -> (173.7104, 514.2029)
  line L4 (244.6953, 493.7615) -> (180.9165, 500.1224)
  arc A3 (173.7104, 508.0829) -> (180.9165, 500.1224) centre (181.7104, 508.0829) ccw
  line L5 (173.7104, 508.0829) -> (173.7104, 514.2029)
  arc A4 (363.7104, -79.6771) -> (356.5044, -71.7166) centre (355.7104, -79.6771) ccw
  line L6 (356.5044, -71.7166) -> (292.7256, -65.3556)
  arc A5 (274.7104, -45.4544) -> (292.7256, -65.3556) centre (294.7104, -45.4544) ccw
  arc A6 (244.6953, -65.3556) -> (262.7104, -45.4544) centre (242.7104, -45.4544) ccw
  line L7 (173.7104, -85.7971) -> (363.7104, -85.7971)
  line L8 (173.7104, -79.6771) -> (173.7104, -85.7971)
  arc A7 (180.9165, -71.7166) -> (173.7104, -79.6771) centre (181.7104, -79.6771) ccw
  line L9 (274.7104, -45.4544) -> (274.7104, 473.8602)
  line L10 (262.7104, 473.8602) -> (262.7104, -45.4544)
  line L11 (244.6953, -65.3556) -> (180.9165, -71.7166)
  point P0 (262.5027, 203.4372)
  point P1 (268.7104, 514.2029)
  point P2 (319.2104, -67.9971)
  point P3 (268.7104, -85.7971)
  dimension "d1225" = 600
  dimension "d1226" = 190
  dimension "d1227" = 12
  dimension "d1228" = 20
  dimension "d1229" = 8
  dimension "d1230" = 6.12
  dimension "d1231" = 44.5
  dimension "d1232" = 17.8
  measures "d1225" distance between parallel lines of L7 L3
  measures "d1226" distance of L8.end L0.start
  measures "d1227" distance between parallel lines of L10 L9
  measures "d1228" radius of A5
  measures "d1229" radius of A4
  measures "d1230" distance of L0.start L0.end
  measures "d1231" horizontal distance of L0.start point (319.21, -67.997)
  measures "d1232" distance from line of L7 point (319.21, -67.997)
sketch "Эскиз5" plane through (0, 0, 0) normal (0, 0, 1) x (1, 0, 0)
  line L0 (-180, 180) -> (180, 180)
  line L1 (180, 180) -> (180, -180)
  line L2 (180, -180) -> (-180, -180)
  line L3 (-180, -180) -> (-180, 180)
  circle A0 centre (-130, 130) radius 18
  circle A1 centre (130, 130) radius 18
  circle A2 centre (130, -130) radius 18
  circle A3 centre (-130, -130) radius 18
  point P0 (0, 0)
  point P1 (0, 180)
  point P2 (-180, 0)
  dimension "d1233" = 360
  dimension "d1234" = 360
  dimension "d1235" = 36
  dimension "d1236" = 130
  dimension "d1237" = 130
  dimension "d1238" = 130
  dimension "d1239" = 130
  constraints: 8 end point, 4 centre point, 3 equal radius, 3 horizontal alignment, 3 vertical alignment, 2 midpoint, 2 parallel, 1 horizontal, 1 perpendicular
  measures "d1233" distance of L2.end L0.start
  measures "d1234" distance of L1.end L2.end
  measures "d1235" diameter of A0
  measures "d1236" horizontal distance of point (0, 0) A0.centre
  measures "d1237" horizontal distance of point (0, 0) A3.centre
  measures "d1238" horizontal distance of point (0, 0) A3.centre
  measures "d1239" horizontal distance of A2.centre point (0, 0)
extrude "Выдавливание1" add sketch "Эскиз5" along normal blind 20
sketch "Эскиз6" plane through (0, 0, 20) normal (0, 0, 1) x (1, 0, 0)
  point P0 (0, 0)
sketch "Эскиз7" plane through (0, 0, 20) normal (0, 0, 1) x (1, 0, 0)
  line L0 (-62.5, 70) -> (62.5, 70)
  line L1 (70, 62.5) -> (70, -62.5)
  line L2 (62.5, -70) -> (-62.5, -70)
  line L3 (-70, -62.5) -> (-70, 62.5)
  arc A0 (-62.5, 70) -> (-70, 62.5) centre (-62.5, 62.5) ccw
  arc A1 (70, 62.5) -> (62.5, 70) centre (62.5, 62.5) ccw
  arc A2 (-70, -62.5) -> (-62.5, -70) centre (-62.5, -62.5) ccw
  arc A3 (62.5, -70) -> (70, -62.5) centre (62.5, -62.5) ccw
  line L4 (62.5, 65) -> (-62.5, 65)
  arc A4 (-62.5, 65) -> (-65, 62.5) centre (-62.5, 62.5) ccw
  line L5 (-65, 62.5) -> (-65, -62.5)
  arc A5 (-65, -62.5) -> (-62.5, -65) centre (-62.5, -62.5) ccw
  line L6 (-62.5, -65) -> (62.5, -65)
  arc A6 (62.5, -65) -> (65, -62.5) centre (62.5, -62.5) ccw
  line L7 (65, -62.5) -> (65, 62.5)
  arc A7 (65, 62.5) -> (62.5, 65) centre (62.5, 62.5) ccw
  point P0 (0, 0)
  point P1 (-70, 70)
  point P2 (70, 70)
  point P3 (-70, -70)
  point P4 (0, 70)
  point P5 (-70, 0)
  dimension "d1242" = 140
  dimension "d1243" = 140
  dimension "d1244" = 7.5
  dimension "d1245" = 5
  constraints: 16 end point, 16 point on circle, 8 centre point, 8 tangent, 6 point on line, 4 parallel, 3 equal radius, 2 midpoint, 2 perpendicular, 1 horizontal, 1 horizontal alignment, 1 vertical alignment, 7 other
  measures "d1242" distance of point (-70, 70) point (70, 70)
  measures "d1243" distance of point (-70, -70) point (-70, 70)
  measures "d1244" radius of A0
  measures "d1245" distance between parallel lines of L0 L4
extrude "Выдавливание2" add sketch "Эскиз7" along normal blind 1610 separate body
sketch "Эскиз8" plane through (0, 0, 1630) normal (0, 0, 1) x (1, 0, 0)
  line L0 (-130, 100) -> (130, 100)
  line L1 (130, 100) -> (130, -100)
  line L2 (130, -100) -> (-130, -100)
  line L3 (-130, -100) -> (-130, 100)
  point P0 (0, 0)
  point P1 (0, 100)
  point P2 (-130, 0)
  dimension "d1248" = 260
  dimension "d1249" = 200
  constraints: 8 end point, 2 midpoint, 2 parallel, 1 horizontal, 1 horizontal alignment, 1 perpendicular, 1 vertical alignment
  measures "d1248" distance between parallel lines of L1 L3
  measures "d1249" distance of L2.end L0.start
extrude "Выдавливание3" add sketch "Эскиз8" along normal blind 10 separate body
equation "\"d875\" = -0.5 * d540 + 0.5 * d537"
